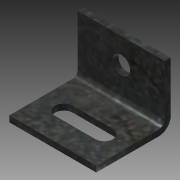
# Autodesk Inventor part: Bracket (15275A53)
Saved by Autodesk Inventor 2015 (Build 190159000, 159)
## iProperties
Created: 2014-05-31
Part Number: Bracket (15275A53)
Material: Steel
Document SubType Name: Sheet Metal
Designer: seaha_000
Density: 7.85 g/cm^3
Sheet Metal Rule: Default
Appearance: Plate
Author: seaha_000
Autodesk Inventor part; units mm, degrees
ref_plane "YZ Plane" through (0, 0, 0) normal (1, 0, 0) x (0, 1, 0)
ref_plane "XZ Plane" through (0, 0, 0) normal (0, 1, 0) x (-1, 0, 0)
ref_plane "XY Plane" through (0, 0, 0) normal (0, 0, 1) x (1, 0, 0)
sketch "Sketch1" plane through (0, 0, 0) normal (0, 1, 0) x (-1, 0, 0)
  line L0 (11.1125, 9.525) -> (-11.1125, 9.525)
  line L1 (-11.1125, 9.525) -> (-11.1125, -9.525)
  line L2 (-11.1125, -9.525) -> (11.1125, -9.525)
  line L3 (11.1125, -9.525) -> (11.1125, 9.525)
  line L4 (11.1125, 9.525) -> (-11.1125, -9.525) construction
  line L5 (-11.1125, 9.525) -> (11.1125, -9.525) construction
  point P0 (0, 0)
  dimension "d0" = 22.225
  dimension "d1" = 19.05
  measures "d0" distance of L1.end L2.end
  measures "d1" distance of L0.end L1.end
extrude "Plate1" add sketch "Sketch1" along normal blind 1.524
sketch "Sketch2" plane through (-11.1125, 0, -8.001) normal (0, 0, -1) x (-1, 0, 0)
  line L0 (-22.225, 0) -> (0, 0)
  line L1 (0, 0) -> (0, 15.875)
  line L2 (0, 15.875) -> (-22.225, 15.875)
  line L3 (-22.225, 15.875) -> (-22.225, 0)
  constraints: 6 end point, 1 horizontal, 1 perpendicular, 1 vertical
edge flange "Flange1" height 15.875 angle 90 thickness 1.524 bend radius 1.524 thickness toward (0, 0, -1) relief tear relief width 1.524 relief depth 0.762 edges at (0, 1.524, -9.525) wall of the first edge with corners at (11.1125, 0, -8.001) (-11.1125, 0, -8.001) (-11.1125, 15.875, -8.001) (11.1125, 15.875, -8.001)
bend "Bend1"
corner "Corner1"
sketch "Sketch3" plane through (0, 1.524, 0) normal (0, 1, 0) x (1, 0, 0)
  line L0 (11.1125, 6.477) -> (-11.1125, 6.477) projected
  line L1 (-11.1125, -9.525) -> (-11.1125, 6.477) projected
  line L2 (11.1125, -9.525) -> (-11.1125, -9.525) projected
  line L3 (11.1125, 6.477) -> (11.1125, -9.525) projected
  line L4 (-11.1125, -1.524) -> (11.1125, -1.524) construction
  line L5 (0, 6.477) -> (0, -9.525) construction
  circle A0 centre (0, -1.524) radius 2.2479
  line L6 (-5.1562, -1.524) -> (5.1562, -1.524) construction
  line L7 (-5.1562, 0.7239) -> (5.1562, 0.7239)
  line L8 (5.1562, -3.7719) -> (-5.1562, -3.7719)
  arc A1 (-5.1562, 0.7239) -> (-5.1562, -3.7719) centre (-5.1562, -1.524) ccw
  arc A2 (5.1562, -3.7719) -> (5.1562, 0.7239) centre (5.1562, -1.524) ccw
  point P0 (0, 0)
  dimension "d13" = 16.002
  dimension "d14" = 22.225
  dimension "d24" = 4.4958
  dimension "d25" = 3.7084
  constraints: 12 end point, 6 midpoint, 5 tangent, 4 point on circle, 3 centre point, 1 horizontal, 1 parallel, 1 point on line, 1 vertical
  measures "d13" diameter of L0 L4
  measures "d14" diameter of L1 L5
  measures "d24" diameter of A0
  measures "d25" distance edge to line of A2 L3
sketch "Sketch4" plane through (-11.1125, 15.875, -8.001) normal (0, 0, 1) x (1, 0, 0)
  line L0 (0, -12.827) -> (22.225, -12.827) projected
  line L1 (22.225, 0) -> (22.225, -12.827) projected
  line L2 (22.225, 0) -> (0, 0) projected
  line L3 (0, 0) -> (0, -12.827) projected
  line L4 (0, -6.4135) -> (22.225, -6.4135) construction
  line L5 (22.225, 0) -> (22.225, -12.827) construction
  line L6 (11.1125, -12.827) -> (11.1125, 0) construction
  line L7 (22.225, 0) -> (0, 0) construction
  point P0 (11.1125, -15.875)
  point P1 (11.1125, -6.4135)
  dimension "d15" = 22.225
  dimension "d16" = 12.827
  constraints: 5 midpoint, 4 end point, 1 perpendicular
  measures "d15" diameter of L1 L6
  measures "d16" diameter of L2 L4
hole "Hole1" at (0, 9.4615, -8.001) direction (0, 0, -1) diameter 4.4958 depth 1.524 tip angle 118 clearance for "Flat Head Machine Screw (82)" size "#8" standard "Ansi Unified Screw Threads"
extrude "Cut1" cut sketch "Sketch3" against normal blind 1.524 contours A0 | A0 L7 A2 L8 | A0 L8 A1 L7
sketch "Sketch7" plane through (11.1125, 15.875, -9.525) normal (0, 0, -1) x (-1, 0, 0)
  line L0 (0, 0) -> (22.225, 0) projected
  line L1 (22.225, -15.875) -> (0, -15.875) projected
  line L2 (0, -12.827) -> (22.225, -12.827) projected
  point P0 (11.1125, -15.875)
  dimension "d28" = 15.875
  dimension "d29" = 12.827
  dimension "d30" = 22.225
  measures "d28" distance between parallel lines of L1 L0
  measures "d29" distance between parallel lines of L2 L0
  measures "d30" distance of L0.start L0.end
sketch "Sketch8" plane through (0, 0, 0) normal (0, -1, 0) x (1, 0, 0)
  arc A0 (-5.1562, 3.7719) -> (-5.1562, -0.7239) centre (-5.1562, 1.524) ccw projected
  line L0 (-5.1562, 3.7719) -> (5.1562, 3.7719) projected
  arc A1 (5.1562, -0.7239) -> (5.1562, 3.7719) centre (5.1562, 1.524) ccw projected
  line L1 (5.1562, -0.7239) -> (-5.1562, -0.7239) projected
  line L2 (-11.1125, -6.477) -> (11.1125, -6.477) projected
  line L3 (11.1125, 9.525) -> (11.1125, -6.477) projected
  line L4 (-11.1125, 9.525) -> (11.1125, 9.525) projected
  line L5 (-11.1125, -6.477) -> (-11.1125, 9.525) projected
  line L6 (11.1125, -9.525) -> (-11.1125, -9.525) projected
  line L7 (11.1125, -6.477) -> (11.1125, -9.525) projected
  line L8 (-11.1125, -6.477) -> (11.1125, -6.477) projected
  line L9 (-11.1125, -9.525) -> (-11.1125, -6.477) projected
  point P0 (0, 0)
  dimension "d31" = 19.05
  dimension "d32" = 16.002
  measures "d31" distance between parallel lines of L6 L4
  measures "d32" distance between parallel lines of L2 L4
sketch "Sketch9" plane through (0, 1.524, 0) normal (0, 1, 0) x (1, 0, 0)
  arc A0 (5.1562, -3.7719) -> (5.1562, 0.7239) centre (5.1562, -1.524) ccw projected
  arc A1 (-5.1562, 0.7239) -> (-5.1562, -3.7719) centre (-5.1562, -1.524) ccw projected
  line L0 (5.1562, -3.7719) -> (-5.1562, -3.7719) projected
  line L1 (-5.1562, 0.7239) -> (5.1562, 0.7239) projected
  circle A2 centre (0, -1.524) radius 2.2479
  point P0 (0, 0)
  dimension "d34" = 5.1562
  constraints: 2 tangent, 1 centre point
  measures "d34" distance of A0.centre A2.centre
sketch "Sketch10" plane through (-11.1125, 15.875, -9.525) normal (0, 1, 0) x (1, 0, 0)
  line L0 (22.225, -19.05) -> (0, -19.05) projected
  line L1 (22.225, 0) -> (0, 0) projected
  line L2 (0, -1.524) -> (0, 0) projected
  line L3 (0, -1.524) -> (0, -3.048) projected
  line L4 (0, -19.05) -> (0, -3.048) projected
  line L5 (0, 0) -> (7.1374, 0)
  line L6 (7.1374, 0) -> (7.1374, -19.05)
  line L7 (7.1374, -19.05) -> (0, -19.05)
  line L8 (0, -19.05) -> (0, 0)
  line L9 (22.225, 0) -> (15.0876, 0)
  line L10 (15.0876, 0) -> (15.0876, -19.05)
  line L11 (15.0876, -19.05) -> (22.225, -19.05)
  line L12 (22.225, -19.05) -> (22.225, 0)
  point P0 (11.1125, -9.525)
  dimension "d35" = 7.1374
  dimension "d36" = 7.1374
  constraints: 16 end point, 4 parallel, 2 horizontal, 2 perpendicular, 2 point on line
  measures "d35" distance between parallel lines of L4 L6
  measures "d36" distance between parallel lines of L12 L10
equation "\"d22\" = Thickness"
equation "\"d26\" = Thickness"
equation "\"d36\" = d35"
equation "\"d3\" = BendReliefWidth"
equation "\"d4\" = BendReliefDepth"
equation "\"d5\" = MinimumRemnant"
equation "\"d6\" = BendRadius"
equation "\"d9\" = BendRadius"
equation "\"d10\" = CornerReliefSize"
equation "\"d11\" = GapSize"
equation "\"d12\" = JacobiRadiusSize"
equation "\"BendRadius\" = Thickness"
equation "\"BendReliefWidth\" = Thickness"
equation "\"BendReliefDepth\" = 0.5 * Thickness"
equation "\"CornerReliefSize\" = 4 * Thickness"
equation "\"MinimumRemnant\" = 2 * Thickness"
equation "\"TransitionRadius\" = BendRadius"
equation "\"JacobiRadiusSize\" = BendRadius"
equation "\"GapSize\" = Thickness"
equation "\"d2\" = BendRadius"
equation "\"Thickness\" = 1.524"
body "Solid1"
